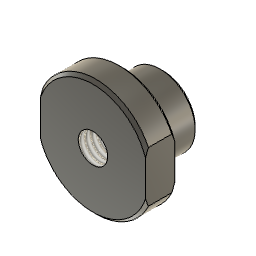
연습예제_3 (Autodesk Fusion 360 design; units mm, degrees)
Autodesk Fusion 360 part; units mm, degrees
sketch "Sketch2" plane through (0, 0, 0) normal (0, 1, 0) x (1, 0, 0)
  circle A0 centre (0, 0) radius 10
  circle A1 centre (0, 0) radius 6
  dimension "d3" = 20
  dimension "d4" = 12
  constraint coincident A0.centre A1.centre
  constraint concentric A0 A1
  measures "d3" diameter of A0
  measures "d4" diameter of A1
extrude "Extrude1" add sketch "Sketch2" along normal blind 5
extrude "Extrude2" add sketch "Sketch2" along normal blind 12 contours A1
hole "Hole1" at (0, 0, 0) direction (0, 1, 0) diameter 5.035 depth 12 tip angle 118
thread "Thread1" "ISO Metric profile 6.0 M6x1 6H"
sketch "Sketch3" plane through (0, 0, 0) normal (0, 1, 0) x (1, 0, 0)
  line L0 (-9, 0) -> (9, 0)
  circle A0 centre (0, 0) radius 10
  line L1 (9, -4.3589) -> (9, 4.3589)
  line L2 (9, 4.3589) -> (12, 4.3589)
  line L3 (12, 4.3589) -> (12, -4.3589)
  line L4 (12, -4.3589) -> (9, -4.3589)
  line L5 (-9, 0) -> (-9, -4.3589)
  line L6 (-9, 0) -> (-9, 4.3589)
  line L7 (-9, 4.3589) -> (-11, 4.3589)
  line L8 (-11, 4.3589) -> (-11, -4.3589)
  line L9 (-11, -4.3589) -> (-9, -4.3589)
  dimension "d12" = 18
  constraint horizontal L0
  constraint midpoint L0 A0.centre
  constraint coincident A0 L1.start
  constraint coincident A0 L1.end
  constraint perpendicular L0 L1
  constraint perpendicular L1 L2
  constraint perpendicular L2 L3
  constraint perpendicular L1 L4
  constraint coincident A0 L5.end
  constraint perpendicular L0 L5
  constraint coincident A0 L6.end
  constraint perpendicular L0 L6
  constraint perpendicular L6 L7
  constraint perpendicular L7 L8
  constraint perpendicular L5 L9
  measures "d12" distance of L0.start L0.end
extrude "Extrude3" cut sketch "Sketch3" along normal through all contours A0 L5 L6 | A0 L1
chamfer "Chamfer1" distance 0.5 angle 45 5 edges at (0, 0, 10) (0, 0, -10) (0, 5, -10) (0, 5, 10) (-5.594, 12, 2.1697)
move_body "Move1" bodies 1 to x (1, 0, 0) y (0, 1, 0) z (0, 0, 1) at (0, 0, 10)
